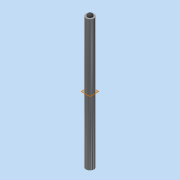
# Autodesk Inventor part: FOX-ME-124
Saved by Autodesk Inventor 2014 (Build 180170000, 170)
## iProperties
Created: 2012-08-10
Part Number: FOX-ME-124
Document SubType Name: Modeling
Designer: Robert Davis
Density: 7.3 g/cm^3
Description: MAGNET
Material: ALNICO5
Mass: 4.40408 g
Surface Area: 4.43369 cm^2
Volume: 0.603299 cm^3
Appearance: Silver
Author: Robert Davis
Autodesk Inventor part; units mm, degrees
ref_plane "YZ Plane" through (0, 0, 0) normal (1, 0, 0) x (0, 1, 0)
ref_plane "XZ Plane" through (0, 0, 0) normal (0, 1, 0) x (-1, 0, 0)
sketch "Sketch1" plane through (0, 0, 0) normal (0, 0, 1) x (1, 0, 0)
  circle A0 centre (0, 0) radius 1.5875
  dimension "d0" = 3.175
  constraints: 1 centre point
  measures "d0" diameter of A0
extrude "Extrusion1" add sketch "Sketch1" along normal mid plane 50.8
sketch "Sketch2" plane through (0, 0, 0) normal (1, 0, 0) x (0, 1, 0)
  line L0 (0, 25.4) -> (0, 26.4)
  line L1 (0, 25.4) -> (1, 25.4)
  arc A0 (1, 25.4) -> (0, 26.4) centre (0, 25.4) ccw
  line L2 (-1.5875, 25.4) -> (1.5875, 25.4) projected
  line L3 (0, 26.4) -> (0, 27.0888)
  point P0 (0, 0)
  dimension "d3" = 1
  constraints: 6 end point, 2 perpendicular, 2 point on circle, 1 centre point, 1 coincident, 1 midpoint, 1 vertical
  measures "d3" radius of A0
revolve "Revolution1" add sketch "Sketch2" angle 360 about axis through (0, 0, 26.4) along (0, 0, 1)
body "Solid1"
